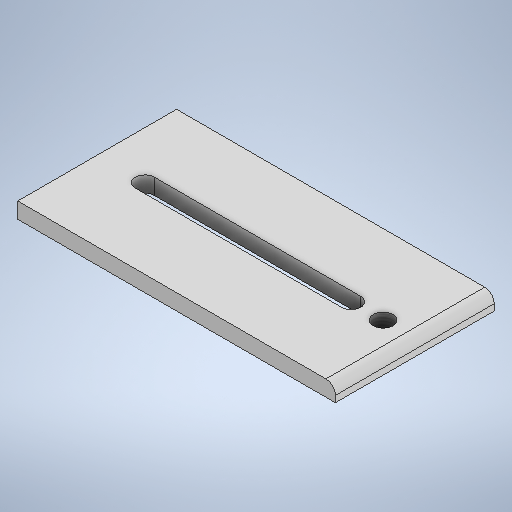
# Autodesk Inventor part: Horonyrogzito
Saved by Autodesk Inventor 2025.2 (Build 292293000, 293)
## iProperties
Created: 2025-08-22
Part Number: Horonyrogzito
Material: Generic
Document SubType Name: Modeling
Designer: MB
Density: 1 g/cm^3
Appearance: Default
Author: MB
Autodesk Inventor part; units mm, degrees
ref_plane "YZ Plane" through (0, 0, 0) normal (1, 0, 0) x (0, 1, 0)
sketch "Sketch1" plane through (0, 0, 0) normal (0, 1, 0) x (-1, 0, 0)
  line L0 (0, 0) -> (-100, 0)
  line L1 (-100, 0) -> (-100, 50)
  line L2 (-100, 50) -> (0, 50)
  line L3 (0, 50) -> (0, 0)
  point P0 (-50, 0)
  point P1 (-90, 25)
  dimension "d0" = 100
  dimension "d1" = 50
  dimension "d24" = 10
  dimension "d25" = 25
  constraints: 8 end point, 2 parallel, 1 horizontal, 1 midpoint, 1 perpendicular
  measures "d0" distance of L1.end L2.end
  measures "d1" distance of L0.end L1.end
  measures "d24" distance from line of L1 point (-90, 25)
  measures "d25" distance from line of point (-90, 25) L2
extrude "Extrusion1" add sketch "Sketch1" along normal blind 5
sketch "Sketch2" plane through (0, 5, 0) normal (0, 1, 0) x (1, 0, 0)
  line L0 (0, -50) -> (100, -50) construction
  line L1 (100, -50) -> (100, 0) construction
  line L2 (100, 0) -> (0, 0) construction
  line L3 (0, 0) -> (0, -50) construction
  line L4 (80, -25) -> (15, -25) construction
  arc A0 (80, -28) -> (80, -22) centre (80, -25) ccw
  arc A1 (15, -22) -> (15, -28) centre (15, -25) ccw
  line L5 (15, -22) -> (80, -22)
  line L6 (80, -28) -> (15, -28)
  point P0 (50, -50)
  dimension "d7" = 65
  dimension "d8" = 25
  dimension "d9" = 15
  dimension "d10" = 6
  dimension "dia" = 6
  constraints: 6 end point, 4 point on circle, 3 tangent, 2 centre point, 2 coincident, 1 horizontal, 1 midpoint
  measures "d7" distance of L4.start L4.end
  measures "d8" distance between parallel lines of L2 L4
  measures "d9" distance from line of L3 L4.end
  measures "d10" diameter of A0
  measures "dia" diameter of A1
extrude "Extrusion2" cut sketch "Sketch2" against normal blind 5
sketch "Sketch5" plane through (0, 5, 0) normal (0, 1, 0) x (1, 0, 0)
  line L0 (0, -50) -> (100, -50) projected
  line L1 (100, -50) -> (100, 0) projected
  point P0 (0, 0)
  point P1 (90, -25)
  dimension "d33" = 25
  dimension "d34" = 10
  measures "d33" distance from line of L0 point (90, -25)
  measures "d34" distance from line of L1 point (90, -25)
hole "Hole1" at (90, 5, 25) direction (0, -1, 0) diameter 6.2 end through all
thread "Thread1" size "M6x1" class "6H" standard "ANSI Metric M Profile" full length
ref_plane "Work Plane1" through (100, 5, 5) normal (0, 0, -1) x (-1, 0, 0)
ref_plane "Work Plane2" through (0, 5, 45) normal (0, 0, 1) x (1, 0, 0)
fillet "Fillet1" radius 3 1 edges at (100, 5, 25)
equation "\"d10\" = dia"
body "Solid1"
